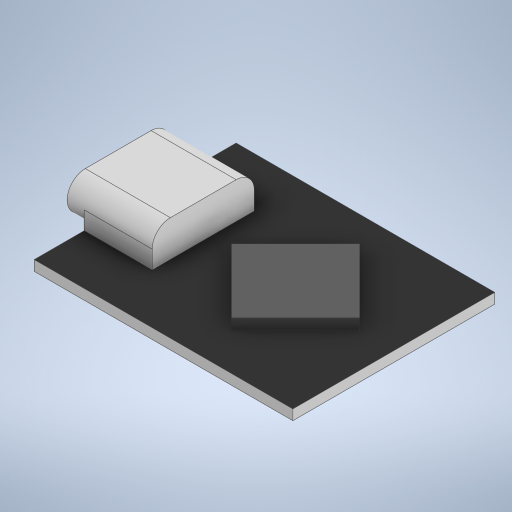
# Autodesk Inventor part: rp2040
Saved by Autodesk Inventor 2023 (Build 270158000, 158)
## iProperties
Created: 2024-03-19
Part Number: rp2040
Material: Generic
Document SubType Name: Modeling
Designer: noname
Density: 1 g/cm^3
Appearance: Default
Author: noname
Autodesk Inventor part; units mm, degrees
ref_plane "YZ Plane" through (0, 0, 0) normal (1, 0, 0) x (0, 1, 0)
ref_plane "XZ Plane" through (0, 0, 0) normal (0, 1, 0) x (-1, 0, 0)
ref_plane "XY Plane" through (0, 0, 0) normal (0, 0, 1) x (1, 0, 0)
sketch "Sketch1" plane through (0, 0, 0) normal (0, 1, 0) x (-1, 0, 0)
  line L0 (0, 0) -> (-22.8, 0)
  line L1 (-22.8, 0) -> (-22.8, -17.8)
  line L2 (-22.8, -17.8) -> (0, -17.8)
  line L3 (0, -17.8) -> (0, 0)
  dimension "d0" = 22.8
  dimension "d1" = 17.8
  constraints: 8 end point, 2 parallel, 1 horizontal, 1 perpendicular
  measures "d0" distance between parallel lines of L1 L3
  measures "d1" distance between parallel lines of L2 L0
extrude "Extrusion1" add sketch "Sketch1" along normal blind 0.9
sketch "Sketch2" plane through (0, 0.9, 0) normal (0, 1, 0) x (1, 0, 0)
  line L0 (14.1431, 3.2431) -> (8.4863, 8.9)
  line L1 (8.4863, 8.9) -> (14.1431, 14.5569)
  line L2 (14.1431, 14.5569) -> (19.8, 8.9)
  line L3 (19.8, 8.9) -> (14.1431, 3.2431)
  line L4 (22.8, 0) -> (22.8, 17.8) projected
  point P0 (0, 0)
  point P1 (22.8, 8.9)
  dimension "d4" = 135
  dimension "d5" = 8
  dimension "d6" = 3
  constraints: 8 end point, 2 parallel, 2 perpendicular, 1 horizontal alignment, 1 midpoint
  measures "d4" angle of L4 L2
  measures "d5" distance between parallel lines of L2 L0
  measures "d6" distance from line of L4 L2.end
extrude "Extrusion2" add sketch "Sketch2" along normal blind 1
sketch "Sketch3" plane through (0, 0.9, 0) normal (0, 1, 0) x (1, 0, 0)
  line L0 (6, 4.4) -> (-1.5, 4.4)
  line L1 (-1.5, 4.4) -> (-1.5, 13.4)
  line L2 (-1.5, 13.4) -> (6, 13.4)
  line L3 (6, 13.4) -> (6, 4.4)
  line L4 (0, 17.8) -> (0, 0) projected
  point P0 (-1.5, 8.9)
  point P1 (0, 8.9)
  dimension "d9" = 7.5
  dimension "d10" = 1.5
  dimension "d11" = 9
  constraints: 8 end point, 2 midpoint, 2 parallel, 1 horizontal, 1 horizontal alignment, 1 perpendicular
  measures "d9" distance between parallel lines of L3 L1
  measures "d10" distance between parallel lines of L4 L1
  measures "d11" distance between parallel lines of L2 L0
extrude "Extrusion3" add sketch "Sketch3" along normal blind 3.2
fillet "Fillet1" radius 1.6 4 edges at (2.25, 4.1, -4.4) (2.25, 4.1, -13.4) (-0.75, 0.9, -4.4) (-0.75, 0.9, -13.4)
body "Solid1"
